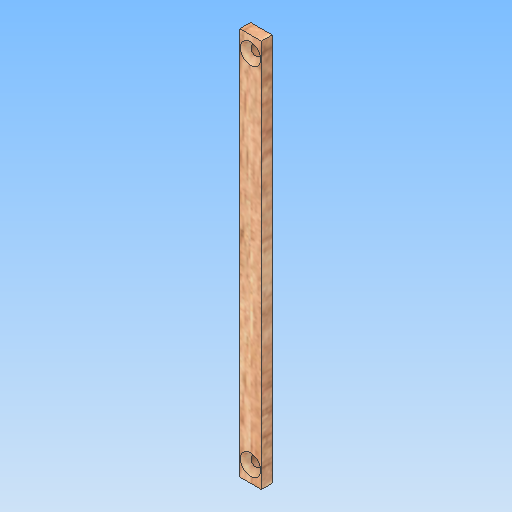
# Autodesk Inventor part: Pancake_Exit Piece
Saved by Autodesk Inventor 2018.1 (Build 221171000, 171)
## iProperties
Created: 2019-02-25
Part Number: Pancake_Exit Piece
Material: Wood (Birch)
Document SubType Name: Modeling
Designer: James
Density: 0.55 g/cm^3
Appearance: Birch - Natural Polished
Mass: 4.79891 g
Surface Area: 55.528 cm^2
Volume: 8.7253 cm^3
Author: James
Autodesk Inventor part; units mm, degrees
ref_plane "YZ Plane" through (0, 0, 0) normal (1, 0, 0) x (0, 1, 0)
ref_plane "XZ Plane" through (0, 0, 0) normal (0, 1, 0) x (-1, 0, 0)
ref_plane "XY Plane" through (0, 0, 0) normal (0, 0, 1) x (1, 0, 0)
sketch "Sketch1" plane through (0, 0, 0) normal (0, 0, 1) x (1, 0, 0)
  line L0 (0, 0) -> (-10, 0)
  line L1 (-10, 0) -> (-10, 180)
  line L2 (-10, 180) -> (0, 180)
  line L3 (0, 180) -> (0, 0)
  dimension "d0" = 10
  dimension "d1" = 180
  constraints: 8 end point, 2 parallel, 1 horizontal, 1 perpendicular
  measures "d0" distance of L0.start L0.end
  measures "d1" distance of L2.end L0.start
extrude "Extrusion1" add sketch "Sketch1" along normal blind 5
sketch "Sketch2" plane through (0, 0, 5) normal (0, 0, 1) x (1, 0, 0)
  line L0 (0, 180) -> (-10, 180) projected
  line L1 (-10, 0) -> (0, 0) projected
  line L2 (-10, 180) -> (-10, 0) projected
  line L3 (0, 0) -> (0, 180) projected
  point P0 (-5, 172.5)
  point P1 (-5, 7.5)
  dimension "d4" = 7.5
  dimension "d5" = 7.5
  dimension "d8" = 5
  dimension "d9" = 5
  constraints: 1 vertical alignment
  measures "d4" distance from line of L0 point (-5, 172.5)
  measures "d5" distance from line of L1 point (-5, 7.5)
  measures "d8" distance from line of L2 point (-5, 172.5)
  measures "d9" distance from line of L3 point (-5, 172.5)
hole "Hole1" at (-5, 172.5, 5) at (-5, 7.5, 5) direction (0, 0, -1) diameter 4.5 end through all countersink diameter 9.4 countersink angle 90 clearance for "Flat Head Machine Screw" size "M4" standard "Ansi Metric M Profile"
equation "\"d5\" = d4"
equation "\"d8\" = d9"
body "Solid1"
